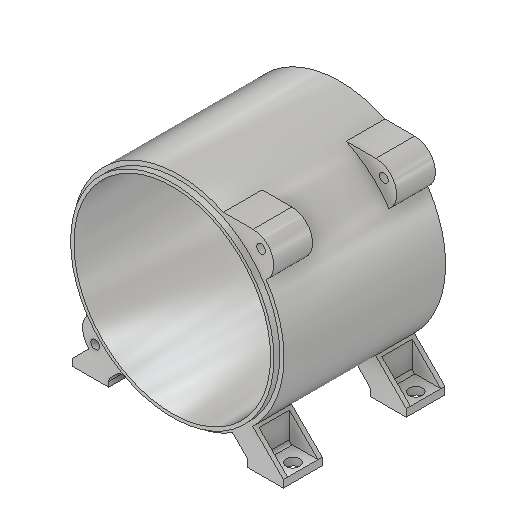
# Autodesk Inventor part: COTS_HP_BLC7000_Fan_Case
Saved by Autodesk Inventor 2026.1 (Build 301233000, 233)
## iProperties
Created: 2020-03-28
Part Number: COTS_HP_BLC7000_Fan_Case
Material: Generic
Document SubType Name: Modeling
Designer: Andrzej
Density: 1 g/cm^3
Appearance: Aluminum - Polished
Author: Andrzej
Autodesk Inventor part; units mm, degrees
ref_plane "YZ Plane" through (0, 0, 0) normal (1, 0, 0) x (0, 1, 0)
sketch "Sketch1" plane through (0, 0, 0) normal (0, 0, 1) x (1, 0, 0)
  circle A0 centre (0, 0) radius 35.5
  circle A1 centre (0, 0) radius 34.1
  circle A2 centre (0, 0) radius 33
  circle A3 centre (0, 0) radius 39.33
  circle A4 centre (27.8105, 27.8105) radius 1.5
  circle A5 centre (-27.8105, -27.8105) radius 1.5
  line L0 (25.1023, 25.1023) -> (27.8105, 27.8105)
  line L1 (-27.8105, -27.8105) -> (-25.1023, -25.1023)
  arc A6 (-29.5399, -19.6887) -> (-19.6887, -29.5399) centre (-25.1023, -25.1023) ccw
  arc A7 (29.5399, 19.6887) -> (19.6887, 29.5399) centre (25.1023, 25.1023) ccw
  circle A8 centre (0, 0) radius 42.5
  line L2 (25.1023, 32.1023) -> (15.1556, 32.1023)
  line L3 (-25.1023, -32.1023) -> (-15.1556, -32.1023)
  dimension "d0" = 71
  dimension "d1" = 68.2
  dimension "d2" = 66
  dimension "d10" = 6.33
  dimension "d13" = 3
  dimension "d14" = 3
  dimension "d20" = 7
  dimension "d21" = 7
  dimension "d26" = 85
  dimension "d27" = 27.8105
  dimension "d28" = 27.8105
  dimension "d29" = 27.8105
  dimension "d30" = 27.8105
  dimension "d60" = 78.66
  constraints: 9 point on circle, 8 centre point, 8 end point, 7 coincident, 2 tangent, 1 horizontal, 1 parallel, 10 other
  measures "d1" diameter of A1
  measures "d2" diameter of A2
  measures "d10" radial gap between concentric circles of A2 A3
  measures "d13" diameter of A4
  measures "d14" diameter of A5
  measures "d20" radius of A7
  measures "d21" radius of A6
  measures "d26" diameter of A8
  measures "d27" horizontal distance of point (0, 0) L0.end
  measures "d28" horizontal distance of point (0, 0) A4.centre
  measures "d29" horizontal distance of point (0, 0) L1.start
  measures "d30" horizontal distance of point (0, 0) L1.start
  measures "d60" diameter of A3
extrude "Extrusion1" add sketch "Sketch1" along normal blind 2 contours A1
extrude "Extrusion2" add sketch "Sketch1" against normal blind 54.2 contours A0 | A1
sketch "Sketch2" plane through (0, 0, -54.2) normal (0, 0, -1) x (-1, 0, 0)
  circle A0 centre (0, 0) radius 34.4
  circle A1 centre (0, 0) radius 35.5 projected
  circle A2 centre (0, 0) radius 33 projected
  dimension "d7" = 68.8
  constraints: 1 centre point, 1 coincident
  measures "d7" diameter of A0
extrude "Extrusion3" cut sketch "Sketch2" against normal blind 2 contours A0
sketch "Sketch4" plane through (0, 0, 0) normal (0, 0, 1) x (1, 0, 0)
  circle A0 centre (0, 0) radius 35.5 projected
  circle A1 centre (0, 0) radius 34.1 projected
  line L0 (-43.8314, -38) -> (48.2304, -38)
  line L1 (23.3, -38) -> (35.3, -38)
  line L2 (35.3, -38) -> (35.3, -35.5)
  line L3 (35.3, -35.5) -> (23.3, -35.5)
  line L4 (23.3, -35.5) -> (23.3, -38)
  line L5 (35.3, -35.5) -> (25.0021, -25.2021)
  line L6 (35.3, -35.5) -> (50.755, -35.5) construction
  line L7 (23.3, -35.5) -> (18.2498, -30.4498)
  line L8 (23.3, -35.5) -> (31.086, -35.5) construction
  dimension "d31" = 38
  dimension "d32" = 12
  dimension "d33" = 2.5
  dimension "d34" = 23.3
  dimension "d36" = 135
  dimension "d38" = 135
  constraints: 18 end point, 4 horizontal, 2 parallel, 2 point on circle, 1 perpendicular, 1 point on line
  measures "d31" distance from line of point (0, 0) L0
  measures "d32" distance of L3.end L2.end
  measures "d33" distance of L2.end L1.end
  measures "d34" distance from line of L4 point (0, 0)
  measures "d36" angle of L6 L5
  measures "d38" angle of L8 L7
extrude "Extrusion7" add sketch "Sketch4" against normal blind 13 contours A0 L5 L3 L7 | L3 L2 L0 L4
ref_plane "Work Plane1" through (23.3, -25, 0) normal (0, -1, 0) x (1, 0, 0)
sketch "Sketch5" plane through (23.3, -25, 0) normal (0, -1, 0) x (1, 0, 0)
  line L0 (0, 0) -> (12, 0) projected
  line L1 (0, 0) -> (0, -13) projected
  line L2 (12, -13) -> (0, -13) projected
  line L3 (12, 0) -> (12, -13) projected
  line L4 (12, 0) -> (12, -13) projected
  line L5 (12, -1.4) -> (2.4, -1.4)
  line L6 (2.4, -1.4) -> (2.4, -11.6)
  line L7 (2.4, -11.6) -> (12, -11.6)
  circle A0 centre (8.7, -6.5) radius 2.25
  point P0 (-23.3, 0)
  dimension "d42" = 9.6
  dimension "d43" = 1.4
  dimension "d44" = 1.4
  dimension "d45" = 4.5
  dimension "d46" = 3.3
  dimension "d47" = 5.1
  dimension "d48" = 10.2
  constraints: 6 end point, 2 perpendicular, 2 point on line, 1 centre point, 1 horizontal
  measures "d42" distance between parallel lines of L3 L6
  measures "d43" distance between parallel lines of L0 L5
  measures "d44" distance between parallel lines of L2 L7
  measures "d45" diameter of A0
  measures "d46" distance from line of L3 A0.centre
  measures "d47" distance from line of L5 A0.centre
  measures "d48" distance of L5.end L6.end
extrude "Extrusion8" cut sketch "Sketch5" along normal blind 10.5 contours L3 L7 L6 L5 | A0
extrude "Extrusion9" cut sketch "Sketch5" along normal up to surface (13 mm away) contours A0
fillet "Fillet2" radius 2 1 edges at (23.3, -35.5, -6.5)
fillet "Fillet2" radius 1 1 edges at (25.7, -35.5, -6.5)
mirror "Mirror1" about plane through (0, 0, 0) normal (1, 0, 0) of "Extrusion7", "Extrusion9", "Extrusion8", "Fillet2"
extrude "Extrusion10" add sketch "Sketch1" against normal blind 13 contours A0 L0 A4 A3 A7 | L3 A3 A6 A0 | A0 A7 A3 A4 L0 | A3 A4 A7 | A6 A3 A5 L1 A0 | L3 A6 A3 | A0 L2 A3 A7 | L0 A3 A4 | A4 A3 L0 | A3 A4 | L1 A5 A3 A6 A0 | A6 A3 A5 | A3 L2 A7 | L1 A3 A5 | A5 A3 L1 | A5 A3
extrude "Extrusion11" cut sketch "Sketch1" against normal blind 13 contours L0 A3 A4 | A4 A3 L0 | A3 A4 | L1 A3 A5 | A5 A3 L1 | A5 A3
ref_plane "Work Plane2" through (0, 0, -27.1) normal (0, 0, 1) x (1, 0, 0)
mirror "Mirror2" about plane through (0, 0, -27.1) normal (0, 0, 1) of "Extrusion7", "Extrusion9", "Extrusion8", "Fillet2", "Mirror1", "Extrusion10", "Extrusion11"
equation "\"d44\" = d43"
equation "\"d47\" = 0.5 * d48"
body "Solid1"
